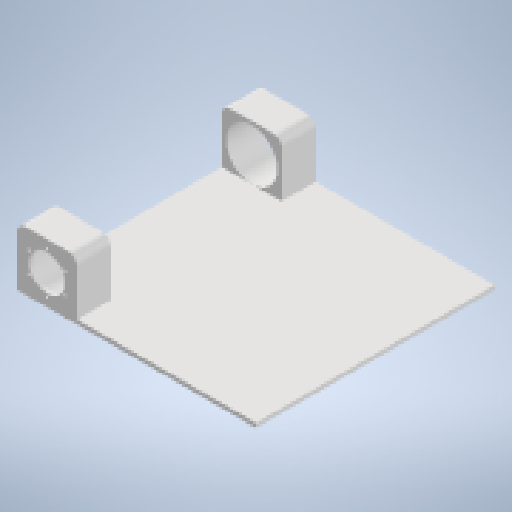
# Autodesk Inventor part: Bot v3
Saved by Autodesk Inventor 2024 (Build 280153000, 153)
## iProperties
Created: 2023-11-20
Part Number: Bot v3
Material: Generic
Document SubType Name: Modeling
Designer: CJ110
Density: 1 g/cm^3
Appearance: Default
Author: CJ110
Autodesk Inventor part; units mm, degrees
ref_plane "YZ Plane" through (0, 0, 0) normal (1, 0, 0) x (0, 1, 0)
ref_plane "XZ Plane" through (0, 0, 0) normal (0, 1, 0) x (-1, 0, 0)
ref_plane "XY Plane" through (0, 0, 0) normal (0, 0, 1) x (1, 0, 0)
sketch "Sketch1" plane through (0, 0, 0) normal (0, 1, 0) x (-1, 0, 0)
  line L0 (177.8, 177.8) -> (0, 177.8)
  line L1 (0, 177.8) -> (0, 0)
  line L2 (0, 0) -> (177.8, 0)
  line L3 (177.8, 0) -> (177.8, 177.8)
  dimension "d0" = 177.8
  dimension "d1" = 177.8
  constraints: 8 end point, 2 parallel, 1 horizontal, 1 perpendicular
  measures "d0" distance of L2.end L0.start
  measures "d1" distance between parallel lines of L1 L3
extrude "Extrusion1" add sketch "Sketch1" along normal blind 3.175
sketch "Sketch2" plane through (0, 3.175, 0) normal (0, 1, 0) x (1, 0, 0)
  line L0 (-177.8, -177.8) -> (0, -177.8) projected
  line L1 (-177.8, -177.8) -> (-133.35, -177.8)
  line L2 (-133.35, -177.8) -> (-133.35, -152.4)
  line L3 (-133.35, -152.4) -> (-177.8, -152.4)
  line L4 (-177.8, -152.4) -> (-177.8, -177.8)
  line L5 (0, 0) -> (-177.8, 0) projected
  line L6 (-177.8, 0) -> (-133.35, 0)
  line L7 (-133.35, 0) -> (-133.35, -25.4)
  line L8 (-133.35, -25.4) -> (-177.8, -25.4)
  line L9 (-177.8, -25.4) -> (-177.8, 0)
  line L10 (-177.8, 0) -> (-177.8, -177.8) projected
  point P0 (-133.35, 0)
  dimension "d4" = 44.45
  dimension "d5" = 25.4
  constraints: 16 end point, 4 parallel, 4 point on line, 2 collinear, 2 horizontal, 2 perpendicular
  measures "d4" distance between parallel lines of L4 L2
  measures "d5" distance of L1.end L2.end
extrude "Extrusion2" add sketch "Sketch2" along normal blind 40.64
sketch "Sketch3" plane through (-177.8, 0, 177.8) normal (0, 0, 1) x (1, 0, 0)
  line L0 (0, 0) -> (177.8, 0) projected
  line L1 (177.8, 0) -> (177.8, 3.175) projected
  line L2 (44.45, 3.175) -> (177.8, 3.175) projected
  line L3 (44.45, 3.175) -> (44.45, 43.815) projected
  line L4 (0, 43.815) -> (44.45, 43.815) projected
  line L5 (0, 0) -> (0, 43.815) projected
  circle A0 centre (22.225, 22.225) radius 19.05
  line L6 (44.45, 3.175) -> (0, 3.175) projected
  line L7 (0, 3.175) -> (44.45, 3.175) projected
  line L8 (44.45, 3.175) -> (177.8, 3.175) projected
  line L9 (177.8, 3.175) -> (44.45, 3.175) projected
  line L10 (22.225, 43.815) -> (22.225, 3.175) construction
  line L11 (0, 0) -> (0, 43.815) projected
  point P0 (177.8, 0)
  dimension "d8" = 38.1
  constraints: 2 end point, 2 midpoint, 1 centre point, 1 point on line, 1 tangent, 1 vertical
  measures "d8" diameter of A0
extrude "Extrusion3" cut sketch "Sketch3" against normal through all contours A0
fillet "Fillet1" radius 6.35 4 edges at (-133.35, 43.815, 165.1) (-177.8, 43.815, 165.1) (-177.8, 43.815, 12.7) (-133.35, 43.815, 12.7)
sketch "Sketch4" plane through (-177.8, 0, 177.8) normal (0, 0, 1) x (1, 0, 0)
  circle A0 centre (22.225, 22.225) radius 19.05 projected
  arc A1 (6.35, 43.815) -> (0, 37.465) centre (6.35, 37.465) ccw projected
  line L0 (0, 0) -> (0, 37.465) projected
  line L1 (0, 0) -> (177.8, 0) projected
  line L2 (177.8, 0) -> (177.8, 3.175) projected
  line L3 (44.45, 3.175) -> (177.8, 3.175) projected
  line L4 (44.45, 3.175) -> (44.45, 37.465) projected
  arc A2 (44.45, 37.465) -> (38.1, 43.815) centre (38.1, 37.465) ccw projected
  line L5 (6.35, 43.815) -> (38.1, 43.815) projected
  circle A3 centre (22.225, 22.225) radius 19.05 projected
  circle A4 centre (22.225, 37.719) radius 1.143
  circle A5 centre (22.225, 22.225) radius 15.494 construction
  circle A6 centre (22.225, 22.225) radius 13.335
  circle A7 centre (8.8068, 29.972) radius 1.143
  circle A8 centre (8.8068, 14.478) radius 1.143
  circle A9 centre (22.225, 6.731) radius 1.143
  circle A10 centre (35.6432, 14.478) radius 1.143
  circle A11 centre (35.6432, 29.972) radius 1.143
  line L6 (6.35, 43.815) -> (38.1, 43.815) projected
  line L7 (22.225, 43.815) -> (22.225, 0)
  point P0 (177.8, 0)
  dimension "d12" = 26.67
  dimension "d15" = 360
  dimension "d19" = 15.494
  dimension "d20" = 2.286
  dimension "d21" = 30.988
  constraints: 7 centre point, 3 point on line, 2 end point, 2 vertical alignment, 1 coincident, 1 midpoint, 1 vertical, 15 other
  measures "d12" diameter of A6
  measures "d19" distance of A0.centre A4.centre
  measures "d20" diameter of A4
  measures "d21" distance of A4.centre A9.centre
extrude "Extrusion4" add sketch "Sketch4" against normal blind 3.175 contours A0 L7 A9 A6 A4 | L7 A4 A6 A9 A0
equation "\"DC_Diameter\" = 36.83"
body "Solid1"
